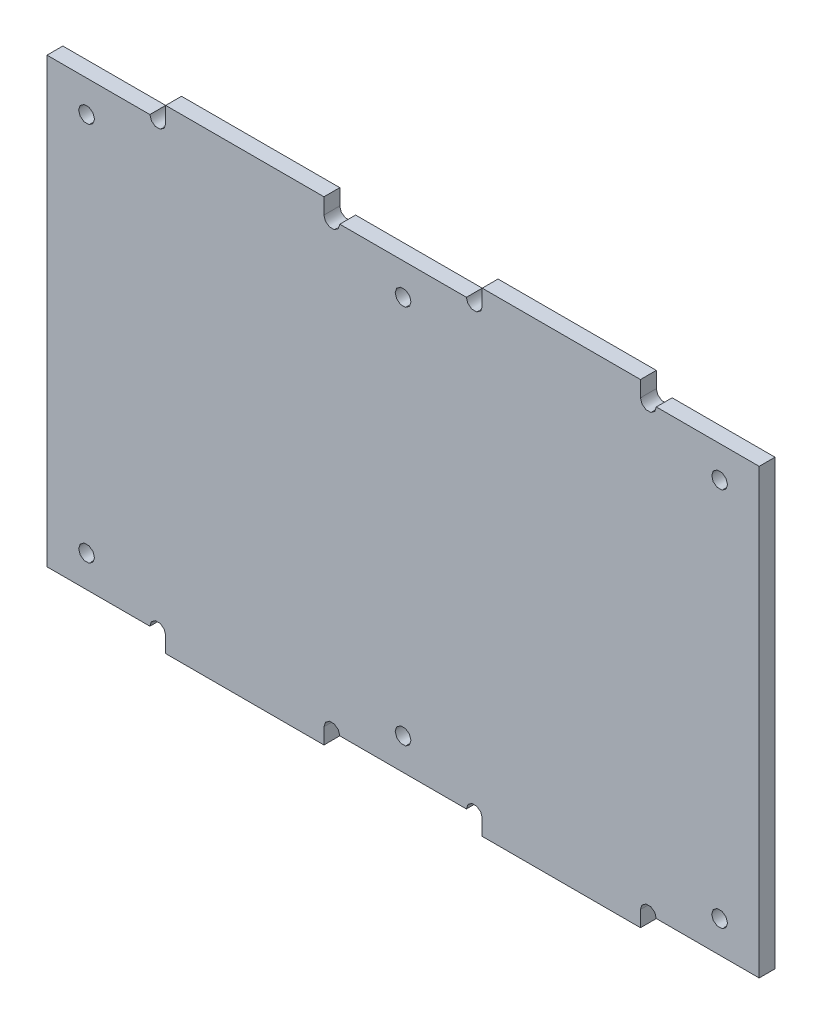
# Autodesk Inventor part: bandeja central
Saved by Autodesk Inventor 2017 (Build 210142000, 142)
## iProperties
Part Number: bandeja central
Material: Genérico
Document SubType Name: Modeling
Designer: Leo
Density: 1 g/cm^3
Appearance: Valor por defecto
Author: Leo
Autodesk Inventor part; units mm, degrees
ref_plane "YZ Plane" through (0, 0, 0) normal (1, 0, 0) x (0, 1, 0)
ref_plane "XZ Plane" through (0, 0, 0) normal (0, 1, 0) x (-1, 0, 0)
ref_plane "XY Plane" through (0, 0, 0) normal (0, 0, 1) x (1, 0, 0)
sketch "Boceto1" plane through (0, 0, 0) normal (0, 0, 1) x (1, 0, 0)
  line L0 (90, 56) -> (90, -56)
  line L1 (90, -56) -> (64, -56)
  arc A0 (64, -56) -> (60, -56) centre (62, -56) ccw
  line L2 (60, -56) -> (60, -60)
  line L3 (60, -60) -> (20, -60)
  line L4 (20, -60) -> (20, -56)
  arc A1 (20, -56) -> (16, -56) centre (18, -56) ccw
  line L5 (15.6321, 0) -> (-15.6321, 0) construction
  line L6 (0, 12.7826) -> (0, -12.7826) construction
  line L7 (90, 56) -> (64, 56)
  arc A2 (60, 56) -> (64, 56) centre (62, 56) ccw
  line L8 (60, 56) -> (60, 60)
  line L9 (60, 60) -> (20, 60)
  line L10 (20, 60) -> (20, 56)
  arc A3 (16, 56) -> (20, 56) centre (18, 56) ccw
  line L11 (-90, 56) -> (-90, -56)
  line L12 (-90, -56) -> (-64, -56)
  arc A4 (-60, -56) -> (-64, -56) centre (-62, -56) ccw
  line L13 (-60, -56) -> (-60, -60)
  line L14 (-60, -60) -> (-20, -60)
  line L15 (-20, -60) -> (-20, -56)
  arc A5 (-16, -56) -> (-20, -56) centre (-18, -56) ccw
  line L16 (-90, 56) -> (-64, 56)
  arc A6 (-64, 56) -> (-60, 56) centre (-62, 56) ccw
  line L17 (-60, 56) -> (-60, 60)
  line L18 (-60, 60) -> (-20, 60)
  line L19 (-20, 60) -> (-20, 56)
  arc A7 (-20, 56) -> (-16, 56) centre (-18, 56) ccw
  line L20 (-16, 56) -> (16, 56)
  line L21 (-16, -56) -> (16, -56)
  circle A8 centre (0, -48) radius 2
  circle A9 centre (0, 48) radius 2
  circle A10 centre (80, 48) radius 2
  circle A11 centre (80, -48) radius 2
  circle A12 centre (-80, 48) radius 2
  circle A13 centre (-80, -48) radius 2
  point P0 (0, 0)
  point P1 (0, 0)
  dimension "d0" = 2
  dimension "d1" = 120
  dimension "d2" = 40
  dimension "d3" = 4
  dimension "d4" = 40
  dimension "d5" = 30
  dimension "d6" = 8
  dimension "d7" = 4
  dimension "d8" = 20
  constraints: 44 end point, 30 symmetric about line, 17 point on line, 16 point on circle, 14 centre point, 4 equal radius, 4 perpendicular, 2 horizontal, 2 horizontal alignment, 2 midpoint, 2 tangent, 2 vertical, 2 vertical alignment, 1 coincident, 1 parallel, 8 other
  measures "d0" radius of A0
  measures "d1" distance between parallel lines of L3 L9
  measures "d2" distance of L2.end L3.end
  measures "d3" distance between parallel lines of L3 L1
  measures "d4" distance between parallel lines of L15 L4
  measures "d5" distance between parallel lines of L0 L2
  measures "d6" distance from line of L20 A9.centre
  measures "d7" diameter of A9
  measures "d8" horizontal distance of L8.end A10.centre
extrude "Extrusión1" add sketch "Boceto1" along normal blind 4
equation "\"d4\" = d2"
